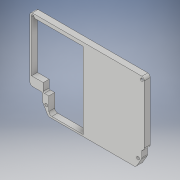
# Autodesk Inventor part: Back Cover
Saved by Autodesk Inventor 2019.4 (Build 234330000, 330)
## iProperties
Created: 2020-08-29
Part Number: Back Cover
Material: Generic
Document SubType Name: Modeling
Designer: craig
Density: 1 g/cm^3
Appearance: Default
Author: craig
## iProperties of the stored document _3DPrint.ipt
Created: 2020-09-02
Part Number: _3DPrint
Material: Generic
Document SubType Name: Modeling
Designer: craig
Density: 1 g/cm^3
Appearance: Default
Author: craig
Autodesk Inventor part; units mm, degrees
ref_plane "YZ Plane" through (0, 0, 0) normal (1, 0, 0) x (0, 1, 0)
ref_plane "XZ Plane" through (0, 0, 0) normal (0, 1, 0) x (-1, 0, 0)
ref_plane "XY Plane" through (0, 0, 0) normal (0, 0, 1) x (1, 0, 0)
sketch "Sketch7" plane through (0, 0, 0) normal (0, 0, 1) x (1, 0, 0)
  line L0 (92.45, -34.85) -> (92.2893, -34.85) projected
  line L1 (92.2893, -34.85) -> (92.2893, -46.3269) projected
  line L2 (92.2893, -46.3269) -> (83.2555, -46.3269) projected
  line L3 (83.2555, -46.3269) -> (83.2555, -34.85) projected
  line L4 (83.2555, -34.85) -> (-64.8533, -34.85) projected
  line L5 (-64.8533, -34.85) -> (-64.8533, -45.8213) projected
  line L6 (-64.8533, -45.8213) -> (-73.8416, -45.8213) projected
  line L7 (-73.8416, -45.8213) -> (-73.8416, -34.85) projected
  line L8 (-73.8416, -34.85) -> (-74.45, -34.85) projected
  line L9 (-74.45, -34.85) -> (-74.45, -19.925) projected
  line L10 (-74.45, -19.925) -> (-94.45, -19.925) projected
  line L11 (-94.45, -19.925) -> (-94.45, 66.85) projected
  line L12 (-94.45, 66.85) -> (-93.95, 66.85) projected
  arc A0 (-90.0713, 69.6192) -> (-93.95, 66.85) centre (-92.45, 68.85) ccw projected
  arc A1 (-90.0713, 69.6192) -> (-86.2653, 66.85) centre (-86.2653, 70.85) ccw projected
  line L13 (-86.2653, 66.85) -> (-73.2725, 66.85) projected
  line L14 (-73.2725, 66.85) -> (-73.2725, 70.4275) projected
  line L15 (-73.2725, 70.4275) -> (92.6104, 70.4275) projected
  arc A2 (95.0772, 66.1658) -> (92.6104, 70.4275) centre (94.2193, 68.514) ccw projected
  arc A3 (95.0772, 66.1658) -> (92.45, 62.4088) centre (96.45, 62.4088) ccw projected
  line L16 (92.45, 62.4088) -> (92.45, -34.85) projected
  arc A4 (98.45, 68.85) -> (94.45, 72.85) centre (94.45, 68.85) ccw projected
  line L17 (94.45, 72.85) -> (-93.45, 72.85) projected
  arc A5 (-93.45, 72.85) -> (-97.45, 68.85) centre (-93.45, 68.85) ccw projected
  line L18 (-97.45, 68.85) -> (-97.45, -35.0582) projected
  line L19 (-97.45, -35.0582) -> (-78, -35.0582) projected
  line L20 (96, -35.0582) -> (98.45, -35.0582) projected
  line L21 (98.45, -35.0582) -> (98.45, 68.85) projected
  arc A6 (-76, -37.0582) -> (-78, -35.0582) centre (-78, -37.0582) ccw projected
  line L22 (-76, -37.0582) -> (-76, -48.5295) projected
  line L23 (-66, -65.85) -> (84, -65.85) projected
  line L24 (94, -48.5295) -> (94, -37.0582) projected
  arc A7 (96, -35.0582) -> (94, -37.0582) centre (96, -37.0582) ccw projected
  circle A8 centre (-69.3475, -50.8213) radius 2.5 projected
  circle A9 centre (87.7724, -50.8213) radius 2.5 projected
  line L25 (94, -48.5295) -> (84, -65.85) projected
  line L26 (-66, -65.85) -> (-76, -48.5295) projected
  point P0 (0, 0)
  point P1 (-74.5366, -65.85)
  point P2 (92.6375, -65.85)
extrude "Extrusion6" add sketch "Sketch7" along normal blind 10 contours L21 L20 A7 L24 L25 L23 L26 L22 A6 L19 L18 A5 L17 A4 | A8 | A9
sketch "Sketch8" plane through (0, 0, 10) normal (0, 0, 1) x (1, 0, 0)
  line L0 (-64.8533, -34.85) -> (83.2555, -34.85)
  line L1 (83.2555, -34.85) -> (83.2555, -62.85)
  line L2 (83.2555, -62.85) -> (-64.8533, -62.85)
  line L3 (-64.8533, -62.85) -> (-64.8533, -34.85)
  line L4 (-66, -65.85) -> (84, -65.85) projected
  point P0 (0, 0)
  point P1 (-76, -65.85)
  point P2 (94, -65.85)
  dimension "d19" = 3
  constraints: 8 end point, 2 coincident, 2 parallel, 1 horizontal, 1 perpendicular
  measures "d19" distance between parallel lines of L4 L2
sketch "Sketch9" plane through (0, 0, 10) normal (0, 0, 1) x (1, 0, 0)
  line L0 (-73.2725, 70.4275) -> (91.6133, 70.4275)
  line L1 (91.6133, 70.4275) -> (91.6133, 67.0798)
  line L2 (91.6133, 67.0798) -> (-73.2725, 67.0798)
  line L3 (-73.2725, 67.0798) -> (-73.2725, 70.4275)
  point P0 (0, 0)
  constraints: 8 end point, 2 parallel, 1 coincident, 1 horizontal, 1 perpendicular
extrude "Extrusion8" add sketch "Sketch9" against normal up to surface (10 mm away)
fillet "Fillet3" radius 2 1 edges at (91.6133, 70.4275, 5)
sketch "Sketch10" plane through (0, 0, 10) normal (0, 0, 1) x (1, 0, 0)
  line L0 (-73.8416, -34.85) -> (-64.8533, -34.85)
  line L1 (-64.8533, -34.85) -> (-64.8533, -45.8213)
  line L2 (-64.8533, -45.8213) -> (-73.8416, -45.8213)
  line L3 (-73.8416, -45.8213) -> (-73.8416, -34.85)
  line L4 (83.2555, -34.85) -> (92.2893, -34.85)
  line L5 (92.2893, -34.85) -> (92.2893, -46.3269)
  line L6 (92.2893, -46.3269) -> (83.2555, -46.3269)
  line L7 (83.2555, -46.3269) -> (83.2555, -34.85)
  point P0 (0, 0)
  constraints: 16 end point, 4 coincident, 4 parallel, 2 horizontal, 2 perpendicular
extrude "Extrusion9" add sketch "Sketch10" against normal up to surface (10 mm away)
extrude "Extrusion10" cut sketch "Sketch8" against normal up to surface (10 mm away)
fillet "Fillet4" radius 5 2 edges at (-64.8533, -62.85, 5) (83.2555, -62.85, 5)
fillet "Fillet4" radius 2 2 edges at (-74.45, -34.85, 5) (92.45, -34.85, 5)
sketch "Sketch11" plane through (0, 0, 10) normal (0, 0, 1) x (1, 0, 0)
  circle A0 centre (-69.3475, -50.8213) radius 2.5 projected
  circle A1 centre (87.7724, -50.8213) radius 2.5 projected
  point P0 (0, 0)
extrude "Extrusion11" cut sketch "Sketch11" against normal up to surface (10 mm away)
fillet "Fillet5" radius 5 6 edges at (98.45, -35.0582, 5) (94, -48.5295, 5) (84, -65.85, 5) (-66, -65.85, 5) (-76, -48.5295, 5) (-97.45, -35.0582, 5)
sketch "Sketch14" plane through (0, 0, 10) normal (0, 0, 1) x (1, 0, 0)
  arc A0 (-97.45, -30.0582) -> (-92.45, -35.0582) centre (-92.45, -30.0582) ccw projected
  line L0 (-92.45, -35.0582) -> (-78, -35.0582) projected
  arc A1 (-76, -37.0582) -> (-78, -35.0582) centre (-78, -37.0582) ccw projected
  line L1 (-76, -37.0582) -> (-76, -47.1897) projected
  arc A2 (-76, -47.1897) -> (-75.3301, -49.6897) centre (-71, -47.1897) ccw projected
  line L2 (-75.3301, -49.6897) -> (-67.4434, -63.35) projected
  arc A3 (-67.4434, -63.35) -> (-63.1132, -65.85) centre (-63.1132, -60.85) ccw projected
  line L3 (-63.1132, -65.85) -> (81.1132, -65.85) projected
  arc A4 (81.1132, -65.85) -> (85.4434, -63.35) centre (81.1132, -60.85) ccw projected
  line L4 (85.4434, -63.35) -> (93.3301, -49.6897) projected
  arc A5 (93.3301, -49.6897) -> (94, -47.1897) centre (89, -47.1897) ccw projected
  line L5 (94, -47.1897) -> (94, -37.0582) projected
  arc A6 (95.2714, -35.1957) -> (94, -37.0582) centre (96, -37.0582) ccw projected
  arc A7 (95.2714, -35.1957) -> (98.45, -30.5392) centre (93.45, -30.5392) ccw projected
  line L6 (98.45, -30.5392) -> (98.45, 68.85) projected
  arc A8 (98.45, 68.85) -> (94.45, 72.85) centre (94.45, 68.85) ccw projected
  line L7 (94.45, 72.85) -> (-93.45, 72.85) projected
  arc A9 (-93.45, 72.85) -> (-97.45, 68.85) centre (-93.45, 68.85) ccw projected
  line L8 (-97.45, 68.85) -> (-97.45, -30.0582) projected
  line L9 (83.2555, -34.85) -> (83.2555, -57.85) projected
  arc A10 (78.2555, -62.85) -> (83.2555, -57.85) centre (78.2555, -57.85) ccw projected
  line L10 (78.2555, -62.85) -> (-59.8533, -62.85) projected
  arc A11 (-64.8533, -57.85) -> (-59.8533, -62.85) centre (-59.8533, -57.85) ccw projected
  line L11 (-64.8533, -57.85) -> (-64.8533, -34.85) projected
  line L12 (-64.8533, -34.85) -> (-72.45, -34.85) projected
  arc A12 (-74.45, -32.85) -> (-72.45, -34.85) centre (-72.45, -32.85) ccw projected
  line L13 (-74.45, -32.85) -> (-74.45, -19.925) projected
  line L14 (-74.45, -19.925) -> (-94.45, -19.925) projected
  line L15 (-94.45, -19.925) -> (-94.45, 66.85) projected
  line L16 (-94.45, 66.85) -> (-93.95, 66.85) projected
  arc A13 (-90.0713, 69.6192) -> (-93.95, 66.85) centre (-92.45, 68.85) ccw projected
  arc A14 (-90.0713, 69.6192) -> (-86.2653, 66.85) centre (-86.2653, 70.85) ccw projected
  line L17 (-86.2653, 66.85) -> (-73.2725, 66.85) projected
  line L18 (-73.2725, 66.85) -> (-73.2725, 67.0798) projected
  line L19 (91.6133, 67.0798) -> (-73.2725, 67.0798) projected
  line L20 (91.6133, 68.6972) -> (91.6133, 67.0798) projected
  arc A15 (92.6104, 70.4275) -> (91.6133, 68.6972) centre (93.6133, 68.6972) ccw projected
  arc A16 (95.0772, 66.1658) -> (92.6104, 70.4275) centre (94.2193, 68.514) ccw projected
  arc A17 (95.0772, 66.1658) -> (92.45, 62.4088) centre (96.45, 62.4088) ccw projected
  line L21 (92.45, 62.4088) -> (92.45, -32.85) projected
  arc A18 (90.45, -34.85) -> (92.45, -32.85) centre (90.45, -32.85) ccw projected
  line L22 (90.45, -34.85) -> (83.2555, -34.85) projected
  circle A19 centre (87.7724, -50.8213) radius 2.5 projected
  circle A20 centre (-69.3475, -50.8213) radius 2.5 projected
  line L23 (-6, 67.0798) -> (-6, -62.85)
  point P0 (0, 0)
  dimension "d36" = 100
  constraints: 2 end point, 2 point on line, 1 perpendicular
  measures "d36" distance between parallel lines of L23 L5
extrude "Extrusion13" add sketch "Sketch14" against normal blind 2 contours L9 A10 L10 L23 L19 L20 A15 A16 A17 L21 A18 L22
sketch "Sketch15" plane through (0, 0, 10) normal (0, 0, 1) x (1, 0, 0)
  arc A0 (95.0772, 66.1658) -> (92.6104, 70.4275) centre (94.2193, 68.514) ccw projected
  arc A1 (92.6104, 70.4275) -> (95.0772, 66.1658) centre (94.2193, 68.514) ccw
  point P0 (0, 0)
  constraints: 2 point on circle, 1 centre point, 1 concentric
extrude "Extrusion14" cut sketch "Sketch15" against normal blind 2
sketch "Sketch16" plane through (-93.45, 72.85, 0) normal (0, 1, 0) x (1, 0, 0)
  line L0 (187.9, 0) -> (0, 0) projected
  line L1 (0, 0) -> (0, -10) projected
  line L2 (187.9, -10) -> (0, -10) projected
  line L3 (187.9, 0) -> (187.9, -10) projected
  point P0 (93.45, 0)
extrude "Extrusion15" add sketch "Sketch16" along normal blind 1
sketch "Sketch17" plane through (0, 0, 0) normal (0, 0, -1) x (-1, 0, 0)
  arc A0 (97.45, 68.85) -> (93.45, 73.85) centre (92.7112, 69.159) ccw
  arc A1 (97.45, 68.85) -> (93.45, 72.85) centre (93.45, 68.85) ccw projected
  line L0 (93.45, 72.85) -> (93.45, 73.85) projected
  arc A2 (-94.45, 73.85) -> (-98.45, 68.85) centre (-93.7112, 69.159) ccw
  arc A3 (-94.45, 72.85) -> (-98.45, 68.85) centre (-94.45, 68.85) ccw projected
  line L1 (-94.45, 72.85) -> (-94.45, 73.85) projected
  point P0 (0, 0)
  constraints: 4 point on circle, 2 centre point, 8 other
extrude "Extrusion16" add sketch "Sketch17" against normal up to surface (10 mm away)
sketch "Sketch18" plane through (-86.2653, 66.85, 0) normal (0, -1, 0) x (1, 0, 0)
  line L0 (80.2653, 8) -> (80.2653, 10) projected
  line L1 (80.2653, 10) -> (12.9929, 10)
  line L2 (177.8786, 0) -> (12.9929, 0)
  line L3 (177.8786, 8) -> (177.8786, 0) projected
  line L4 (177.8786, 8) -> (80.2653, 8) projected
  line L5 (12.9929, 0) -> (0, 0)
  line L6 (0, 10) -> (12.9929, 10)
  line L7 (0, 0) -> (-5.6221, 0)
  line L8 (-5.6221, 0) -> (-5.6221, 10)
  line L9 (-5.6221, 10) -> (0, 10)
  point P0 (86.2653, 0)
  constraints: 14 end point, 1 horizontal, 1 parallel, 1 perpendicular
extrude "Extrusion17" cut sketch "Sketch18" against normal blind 1
sketch "Sketch20" plane through (-94.45, 66.85, 0) normal (0, -1, 0) x (1, 0, 0)
  line L0 (0.5, 0) -> (0, 0) projected
  line L1 (0.5, 0) -> (0.5, 10) projected
  line L2 (0, 10) -> (0.5, 10) projected
  line L3 (0, 0) -> (0, 10) projected
  point P0 (94.45, 0)
extrude "Extrusion19" cut sketch "Sketch20" against normal blind 3
body "Solid4"
